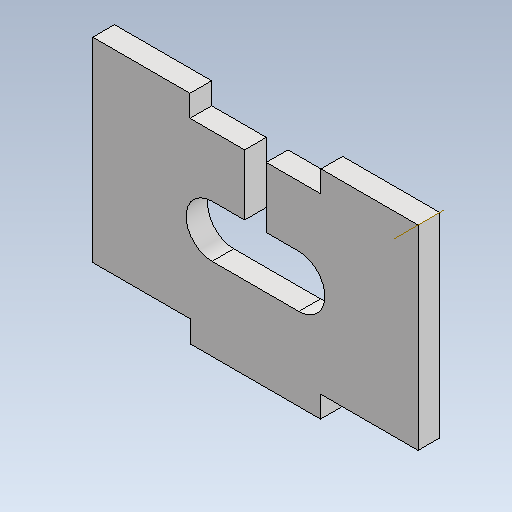
# Autodesk Inventor part: upper-back-plate-support
Saved by Autodesk Inventor 2025 (Build 290162000, 162)
## iProperties
Created: 2025-08-21
Part Number: upper-back-plate-support
Material: Generic
Document SubType Name: Modeling
Designer: HP
Density: 1 g/cm^3
Appearance: Default
Author: HP
Autodesk Inventor part; units mm, degrees
ref_plane "YZ Plane" through (0, 0, 0) normal (1, 0, 0) x (0, 1, 0)
ref_plane "XZ Plane" through (0, 0, 0) normal (0, 1, 0) x (-1, 0, 0)
ref_plane "XY Plane" through (0, 0, 0) normal (0, 0, 1) x (1, 0, 0)
sketch "Sketch1" plane through (0, 0, 0) normal (0, 0, 1) x (1, 0, 0)
  line L0 (-37.5, -25) -> (37.5, -25)
  line L1 (37.5, -25) -> (37.5, 25)
  line L2 (37.5, 25) -> (-37.5, 25)
  line L3 (-37.5, 25) -> (-37.5, -25)
  line L4 (-37.5, -25) -> (37.5, 25) construction
  line L5 (37.5, -25) -> (-37.5, 25) construction
  line L6 (-15.1, 25) -> (15.1, 25)
  line L7 (15.1, 25) -> (15.1, 20)
  line L8 (15.1, 20) -> (-15.1, 20)
  line L9 (-15.1, 20) -> (-15.1, 25)
  line L10 (-15.1, 25) -> (15.1, 20) construction
  line L11 (15.1, 25) -> (-15.1, 20) construction
  line L12 (-4.9474, -25) -> (-37.5, -25)
  line L13 (-37.5, -25) -> (-37.5, -21.6221)
  line L14 (74.3708, -25) -> (124.7526, -25)
  line L15 (0, 0) -> (0, -25) construction
  line L16 (24.4526, -25) -> (37.5, -25)
  line L17 (37.5, -25) -> (37.5, -19.8)
  line L18 (-10, 0) -> (10, 0) construction
  line L19 (-10, -6) -> (10, -6)
  line L20 (10, 6) -> (-10, 6)
  arc A0 (-10, 6) -> (-10, -6) centre (-10, 0) ccw
  arc A1 (10, -6) -> (10, 6) centre (10, 0) ccw
  line L21 (-2.5, 6) -> (2.5, 6)
  line L22 (2.5, 6) -> (2.5, 20)
  line L23 (2.5, 20) -> (-2.5, 20)
  line L24 (-2.5, 20) -> (-2.5, 6)
  line L25 (-2.5, 6) -> (2.5, 20) construction
  line L26 (2.5, 6) -> (-2.5, 20) construction
  line L27 (-37.5, -25) -> (-20.5763, -25)
  line L28 (-37.5, -20) -> (-37.5, -25)
  line L29 (20.5763, -25) -> (37.5, -25)
  line L30 (37.5, -25) -> (37.5, -20)
  line L31 (-15, -25) -> (15, -25)
  line L32 (15, -25) -> (15, -20)
  line L33 (15, -20) -> (-15, -20) construction
  line L34 (-15, -20) -> (-15, -25)
  line L35 (-15, -25) -> (15, -20) construction
  line L36 (15, -25) -> (-15, -20) construction
  line L37 (-15, -20) -> (-37.5, -20)
  line L38 (15, -20) -> (37.5, -20)
  point P0 (0, 22.5)
  point P1 (15.1, 25)
  point P2 (-15.1, 25)
  point P3 (0, 13)
  point P4 (2.5, 20)
  point P5 (0, -22.5)
  dimension "d1" = 50
  dimension "d10" = 5
  dimension "d11" = 30.2
  dimension "d25" = 12
  dimension "d26" = 20
  dimension "d27" = 5
  dimension "d35" = 5
  dimension "d36" = 30
  dimension "d37" = 75
  constraints: 80 end point, 13 collinear, 10 equal length, 10 horizontal, 10 midpoint, 6 perpendicular, 4 point on circle, 4 tangent, 3 vertical alignment, 2 centre point, 1 coincident
  measures "d1" distance between parallel lines of L0 L2
  measures "d10" distance between parallel lines of L8 L6
  measures "d11" distance between parallel lines of L9 L7
  measures "d25" distance between parallel lines of L20 L19
  measures "d26" distance of L18.start L18.end
  measures "d27" distance between parallel lines of L24 L22
  measures "d35" distance between parallel lines of L31 L33
  measures "d36" distance between parallel lines of L32 L34
  measures "d37" distance between parallel lines of L1 L3
extrude "Extrusion1" add sketch "Sketch1" along normal blind 5 contours L34 L37 L3 L2 L9 L8 L24 L20 A0 L19 A1 L22 L7 L1 L38 L32 L0
body "Solid1"
